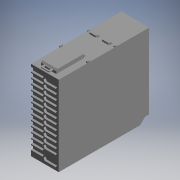
# Autodesk Inventor part: 2247681 CACN-3A-1-5
Saved by Autodesk Inventor 2017.3 (Build 213256000, 256)
## iProperties
Part Number: 2247681 CACN-3A-1-5
Material: Generic
Catalog Web Link: www.cadenas.de
Description: CACN-Power supply unit
Vendor: FESTO
Document SubType Name: Modeling
Designer: partserver
Manufacturer: FESTO
Mass: 600 g
Surface Area: 578.959 cm^2
Volume: 583.76 cm^3
Density: 1 g/cm^3
Appearance: PSOLRGB-175-175-175
Category: PARTsolutions
Company: FESTO
Title: 2247681 CACN-3A-1-5
Author: Cadenas PARTsolutions
Comments: Power supply unit
PSOL_IDENT_0: {$CADENAS_DATA\23d-libs\festo\parts\c\cacn\cacn.prj},176 {VTYP=3D},{NB=2247681 CACN-3A-1-5},{LINA=22
PSOL_IDENT_1: 47681 CACN-3A-1-5},{NN=CACN},{DATE=26.01.2021 14:46:32},{GEOMDATE=19.09.2018 12:21:51},{VERSION=},{L
PSOL_IDENT_2: INEID=50},{WBVAR=},{WBNUMERIC=}  {NB=2247681 CACN-3A-1-5},{LINA=2247681 CACN-3A-1-5},{KT=DUMMY},{TNR=
PSOL_IDENT_3: 2247681},{TYP=CACN-3A-1-5},{A=40.000},{B=130.000},{C=115.000},{VERS=1.000},{CNSMASSEXACT=0.600}
NB: 2247681 CACN-3A-1-5
NN: CACN
NT: Power supply unit
NBSYN: $TNR. $TYP.
LINA: 2247681 CACN-3A-1-5
CATALOG: Festo
TNR: 2247681
TYP: CACN-3A-1-5
A: 40
B: 130
C: 115
CNSMASSEXACT: 0.6
SUPPLIER: FESTO
ARTICLENO: 2247681 CACN-3A-1-5
BOMINFO: 2247681 CACN-3A-1-5
CREATOR: CADENAS GmbH
Autodesk Inventor part; units mm, degrees
ref_plane "YZ Plane" through (0, 0, 0) normal (1, 0, 0) x (0, 1, 0)
ref_plane "XZ Plane" through (0, 0, 0) normal (0, 1, 0) x (-1, 0, 0)
ref_plane "XY Plane" through (0, 0, 0) normal (0, 0, 1) x (1, 0, 0)
sketch "Sketch_1" plane through (0, 0, 0) normal (1, 0, 0) x (0, 1, 0)
  line L0 (52, 115) -> (-65, 115)
  line L1 (-65, 115) -> (-65, 0)
  line L2 (-65, 0) -> (-24, 0)
  line L3 (-24, 0) -> (-24, -2)
  line L4 (-24, -2) -> (-20, -2)
  line L5 (-20, -2) -> (-20, 0)
  line L6 (-20, 0) -> (15.7, 0)
  line L7 (15.7, 0) -> (15.7, -1.36)
  line L8 (15.7, -1.36) -> (18.8, -1.36)
  line L9 (18.8, -1.36) -> (18.8, 0)
  line L10 (18.8, 0) -> (65, 0)
  line L11 (65, 0) -> (65, 108)
  line L12 (65, 108) -> (59, 108)
  line L13 (59, 108) -> (52, 115)
  constraints: 28 end point
extrude "Extrusion1" add sketch "Sketch_1" along normal mid plane 40
sketch "Sketch_2" plane through (0, 0, 0) normal (1, 0, 0) x (0, 1, 0)
  line L0 (-59.6, 3) -> (-59.6, -2.3)
  line L1 (-59.6, -2.3) -> (-65.1, -2.3)
  line L2 (-65.1, -2.3) -> (-65.1, -3.3)
  line L3 (-65.1, -3.3) -> (-59.6, -3.3)
  line L4 (-59.6, -3.3) -> (-57.6, -5.3)
  line L5 (-57.6, -5.3) -> (-20.9073, -5.3)
  arc A0 (-20.9073, -5.3) -> (-20.151, -4.9542) centre (-20.9073, -4.3) ccw
  line L6 (-20.151, -4.9542) -> (-17.3487, -1.7146)
  arc A1 (-17.3487, -1.7146) -> (-17.3, -1.5838) centre (-17.5, -1.5838) ccw
  line L7 (-17.3, -1.5838) -> (-17.3, -1.4748)
  arc A2 (-17.3, -1.4748) -> (-17.473, -1.2766) centre (-17.5, -1.4748) ccw
  line L8 (-17.473, -1.2766) -> (-19.5, -1)
  line L9 (-19.5, -1) -> (-19.5, 0)
  line L10 (-19.5, 0) -> (15.7, 0)
  line L11 (15.7, 0) -> (15.7, -0.85)
  arc A3 (15.11, -1.18) -> (15.7, -0.85) centre (14.9456, -0.1936) ccw
  line L12 (15.11, -1.18) -> (12.47, -1.6455)
  line L13 (12.47, -1.6455) -> (12.8173, -3.6151)
  line L14 (12.8173, -3.6151) -> (15.42, -3.1562)
  arc A4 (15.42, -3.1562) -> (17.71, -1.36) centre (14.9459, -0.1939) ccw
  line L15 (17.71, -1.36) -> (18.8, -1.36)
  line L16 (18.8, -1.36) -> (18.8, 3)
  line L17 (18.8, 3) -> (-59.6, 3)
  constraints: 36 end point, 10 point on circle, 5 centre point
extrude "Extrusion2" add sketch "Sketch_2" along normal mid plane 27
sketch "Sketch_3" plane through (0, 0, 0) normal (0, 0, 1) x (1, 0, 0)
  line L0 (-18, 25) -> (-18, -70)
  line L1 (-18, -70) -> (19, -70)
  line L2 (19, -70) -> (19, 25)
  line L3 (19, 25) -> (-18, 25)
  line L4 (4.65, 20) -> (4.65, 11)
  line L5 (4.65, 11) -> (13.5, 11)
  line L6 (13.5, 11) -> (13.5, 20)
  line L7 (13.5, 20) -> (4.65, 20)
  line L8 (-11, -14.6) -> (-11, -59.6)
  line L9 (-11, -59.6) -> (-6.5, -59.6)
  line L10 (-6.5, -59.6) -> (-6.5, -64.1)
  line L11 (-6.5, -64.1) -> (-5.5, -65.1)
  line L12 (-5.5, -65.1) -> (5.5, -65.1)
  line L13 (5.5, -65.1) -> (6.5, -64.1)
  line L14 (6.5, -64.1) -> (6.5, -59.6)
  line L15 (6.5, -59.6) -> (11, -59.6)
  line L16 (11, -59.6) -> (11, -14.6)
  line L17 (11, -14.6) -> (-11, -14.6)
  line L18 (-13.5, 20) -> (-13.5, 11)
  line L19 (-13.5, 11) -> (-4.65, 11)
  line L20 (-4.65, 11) -> (-4.65, 20)
  line L21 (-4.65, 20) -> (-13.5, 20)
  constraints: 44 end point
extrude "Extrusion3" cut sketch "Sketch_3" against normal blind 8
sketch "Sketch_4" plane through (0, 0, 0) normal (0, 0, 1) x (1, 0, 0)
  line L0 (-4, -60.6) -> (-4, -63.1)
  line L1 (-4, -63.1) -> (4, -63.1)
  line L2 (4, -63.1) -> (4, -60.6)
  line L3 (4, -60.6) -> (-4, -60.6)
  constraints: 8 end point
extrude "Extrusion4" cut sketch "Sketch_4" against normal blind 8
sketch "Sketch_5" plane through (0, 0, 115) normal (0, 0, 1) x (1, 0, 0)
  line L0 (-13.9, 48.5) -> (-13.9, 21)
  line L1 (-13.9, 21) -> (0.4, 21)
  line L2 (0.4, 21) -> (0.4, 48.5)
  line L3 (0.4, 48.5) -> (-13.9, 48.5)
  constraints: 8 end point
extrude "Extrusion5" cut sketch "Sketch_5" against normal blind 3
sketch "Sketch_7" plane through (0, 0, 115) normal (0, 0, 1) x (1, 0, 0)
  line L0 (-13.9, -23.5) -> (-13.9, -48.5)
  line L1 (-13.9, -48.5) -> (0.4, -48.5)
  line L2 (0.4, -48.5) -> (0.4, -23.5)
  line L3 (0.4, -23.5) -> (-13.9, -23.5)
  constraints: 8 end point
sketch "Sketch7" plane through (-20, -65, 115) normal (0, 0, 1) x (1, 0, 0)
  point P0 (11.7, 77.5)
hole "Hole1" at (-8.3, 12.5, 115) direction (0, 0, -1) diameter 4 depth 3
extrude "Extrusion6" cut sketch "Sketch_7" against normal blind 3
sketch "Sketch8" plane through (-20, -65, 115) normal (0, 0, 1) x (1, 0, 0)
  point P0 (11.7, 67.5)
hole "Hole2" at (-8.3, 2.5, 115) direction (0, 0, -1) diameter 4 depth 3
sketch "Sketch_9" plane through (0, 0, 115) normal (0, 0, 1) x (1, 0, 0)
  arc A0 (-19, -63.5) -> (-18.5, -64) centre (-18.5, -63.5) ccw
  line L0 (-18.5, -64) -> (18.5, -64)
  arc A1 (18.5, -64) -> (19, -63.5) centre (18.5, -63.5) ccw
  line L1 (19, -63.5) -> (19, 50.5)
  arc A2 (19, 50.5) -> (18.5, 51) centre (18.5, 50.5) ccw
  line L2 (18.5, 51) -> (-18.5, 51)
  arc A3 (-18.5, 51) -> (-19, 50.5) centre (-18.5, 50.5) ccw
  line L3 (-19, 50.5) -> (-19, -63.5)
  circle A4 centre (-8.3, 2.5) radius 2
  circle A5 centre (-8.3, 12.5) radius 2
  line L4 (-14.4, 49) -> (-14.4, 20.5)
  line L5 (-14.4, 20.5) -> (0.65, 20.5)
  line L6 (0.65, 20.5) -> (0.65, 49)
  line L7 (0.65, 49) -> (-14.4, 49)
  line L8 (-14.4, -23) -> (-14.4, -49)
  line L9 (-14.4, -49) -> (0.65, -49)
  line L10 (0.65, -49) -> (0.65, -23)
  line L11 (0.65, -23) -> (-14.4, -23)
  constraints: 24 end point, 8 point on circle, 6 centre point
extrude "Extrusion7" add sketch "Sketch_9" along normal blind 0.2
sketch "Sketch_10" plane through (0, 0, 112) normal (0, 0, 1) x (1, 0, 0)
  circle A0 centre (-8.3, 12.5) radius 1.5
  constraints: 1 centre point
extrude "Extrusion8" add sketch "Sketch_10" along normal blind 3.5
sketch "Sketch_11" plane through (0, 21, 0) normal (0, 1, 0) x (1, 0, 0)
  arc A0 (-13.9, -114.1) -> (-12.4, -115.6) centre (-12.4, -114.1) ccw
  line L0 (-12.4, -115.6) -> (0, -115.6)
  arc A1 (0, -115.6) -> (0.4, -115.2) centre (0, -115.2) ccw
  line L1 (0.4, -115.2) -> (0.4, -112)
  line L2 (0.4, -112) -> (-13.9, -112)
  line L3 (-13.9, -112) -> (-13.9, -114.1)
  constraints: 8 end point, 4 point on circle, 2 centre point
extrude "Extrusion9" add sketch "Sketch_11" along normal blind 27.5
sketch "Sketch_12" plane through (0, 46, 0) normal (0, 1, 0) x (1, 0, 0)
  line L0 (-11, -110.5) -> (-11, -115.6)
  line L1 (-11, -115.6) -> (-4.6, -115.6)
  line L2 (-4.6, -115.6) -> (-6.85, -111.7029)
  line L3 (-6.85, -111.7029) -> (-6.85, -110.5)
  line L4 (-6.85, -110.5) -> (-11, -110.5)
  constraints: 10 end point
extrude "Extrusion10" cut sketch "Sketch_12" along normal mid plane 4
pattern_linear "Rectangular Pattern1" count 5 spacing 5 along (0, -1, 0) of "Extrusion10"
sketch "Sketch_13" plane through (0, 0, 115.6) normal (0, 0, 1) x (1, 0, 0)
  circle A0 centre (-1.9, 45.75) radius 1.8
  constraints: 1 centre point
extrude "Extrusion11" cut sketch "Sketch_13" along normal mid plane 6
pattern_linear "Rectangular Pattern2" count 5 spacing 5 along (0, -1, 0) of "Extrusion11"
sketch "Sketch_16" plane through (0, -48.5, 0) normal (0, 1, 0) x (1, 0, 0)
  arc A0 (-13.9, -114.1) -> (-12.4, -115.6) centre (-12.4, -114.1) ccw
  line L0 (-12.4, -115.6) -> (0, -115.6)
  arc A1 (0, -115.6) -> (0.4, -115.2) centre (0, -115.2) ccw
  line L1 (0.4, -115.2) -> (0.4, -112)
  line L2 (0.4, -112) -> (-13.9, -112)
  line L3 (-13.9, -112) -> (-13.9, -114.1)
  constraints: 8 end point, 4 point on circle, 2 centre point
extrude "Extrusion12" add sketch "Sketch_16" along normal blind 25
sketch "Sketch_17" plane through (0, -28.5, 0) normal (0, 1, 0) x (1, 0, 0)
  line L0 (-11, -110.5) -> (-11, -115.6)
  line L1 (-11, -115.6) -> (-4.6, -115.6)
  line L2 (-4.6, -115.6) -> (-6.85, -111.7029)
  line L3 (-6.85, -111.7029) -> (-6.85, -110.5)
  line L4 (-6.85, -110.5) -> (-11, -110.5)
  constraints: 10 end point
extrude "Extrusion13" cut sketch "Sketch_17" along normal mid plane 4
pattern_linear "Rectangular Pattern3" count 3 spacing 7.5 along (0, -1, 0) of "Extrusion13"
sketch "Sketch16" plane through (-12.4, -48.5, 115.6) normal (0, 0, 1) x (1, 0, 0)
  point P0 (10.5, 19.75)
hole "Hole3" at (-1.9, -28.75, 115.6) direction (0, 0, -1) diameter 3.6 depth 3
pattern_linear "Rectangular Pattern4" count 3 spacing 7.5 along (0, -1, 0) of "Hole3"
sketch "Sketch_21" plane through (0, 65, 0) normal (0, 1, 0) x (1, 0, 0)
  line L0 (-17.567, -10.5) -> (-15.8349, -13.5)
  line L1 (-15.8349, -13.5) -> (0.2009, -13.5)
  line L2 (0.2009, -13.5) -> (1.933, -10.5)
  line L3 (1.933, -10.5) -> (0.2009, -7.5)
  line L4 (0.2009, -7.5) -> (-15.8349, -7.5)
  line L5 (-15.8349, -7.5) -> (-17.567, -10.5)
  constraints: 12 end point
extrude "Extrusion14" cut sketch "Sketch_21" against normal blind 3
pattern_linear "Rectangular Pattern5" count 11 spacing 7.5 along (0, 0, 1) of "Extrusion14"
sketch "Sketch_25" plane through (0, 65, 0) normal (0, 1, 0) x (1, 0, 0)
  line L0 (-17.567, -100.5) -> (-15.8349, -103.5)
  line L1 (-15.8349, -103.5) -> (0.2009, -103.5)
  line L2 (0.2009, -103.5) -> (1.933, -100.5)
  line L3 (1.933, -100.5) -> (0.2009, -97.5)
  line L4 (0.2009, -97.5) -> (-15.8349, -97.5)
  line L5 (-15.8349, -97.5) -> (-17.567, -100.5)
  constraints: 12 end point
extrude "Extrusion15" cut sketch "Sketch_25" against normal blind 3
sketch "Sketch_26" plane through (0, 65, 0) normal (0, 1, 0) x (1, 0, 0)
  line L0 (1.4, -6.75) -> (3.1321, -9.75)
  line L1 (3.1321, -9.75) -> (20, -9.75)
  line L2 (20, -9.75) -> (20, -3.75)
  line L3 (20, -3.75) -> (3.1321, -3.75)
  line L4 (3.1321, -3.75) -> (1.4, -6.75)
  constraints: 10 end point
extrude "Extrusion16" cut sketch "Sketch_26" against normal blind 3
pattern_linear "Rectangular Pattern6" count 13 spacing 7.5 along (0, 0, 1) of "Extrusion16"
sketch "Sketch_22" plane through (0, -62, 0) normal (0, 1, 0) x (1, 0, 0)
  line L0 (-17.567, -10.5) -> (-15.8349, -13.5)
  line L1 (-15.8349, -13.5) -> (0.2009, -13.5)
  line L2 (0.2009, -13.5) -> (1.933, -10.5)
  line L3 (1.933, -10.5) -> (0.2009, -7.5)
  line L4 (0.2009, -7.5) -> (-15.8349, -7.5)
  line L5 (-15.8349, -7.5) -> (-17.567, -10.5)
  constraints: 12 end point
extrude "Extrusion17" cut sketch "Sketch_22" against normal blind 3
pattern_linear "Rectangular Pattern7" count 12 spacing 7.5 along (0, 0, 1) of "Extrusion17"
sketch "Sketch_28" plane through (0, -62, 0) normal (0, 1, 0) x (1, 0, 0)
  line L0 (-17.567, -108) -> (-15.8349, -111)
  line L1 (-15.8349, -111) -> (0.2009, -111)
  line L2 (0.2009, -111) -> (1.933, -108)
  line L3 (1.933, -108) -> (0.2009, -105)
  line L4 (0.2009, -105) -> (-15.8349, -105)
  line L5 (-15.8349, -105) -> (-17.567, -108)
  constraints: 12 end point
extrude "Extrusion18" cut sketch "Sketch_28" against normal blind 3
sketch "Sketch_29" plane through (0, -62, 0) normal (0, 1, 0) x (1, 0, 0)
  line L0 (1.4, -6.75) -> (3.1321, -9.75)
  line L1 (3.1321, -9.75) -> (20, -9.75)
  line L2 (20, -9.75) -> (20, -3.75)
  line L3 (20, -3.75) -> (3.1321, -3.75)
  line L4 (3.1321, -3.75) -> (1.4, -6.75)
  constraints: 10 end point
extrude "Extrusion19" cut sketch "Sketch_29" against normal blind 3
pattern_linear "Rectangular Pattern8" count 14 spacing 7.5 along (0, 0, 1) of "Extrusion19"
ref_plane "LINKS_XY" through (-20, 0, 0) normal (1, 0, 0) x (0, 1, 0)
ref_plane "LINKS_YZ" through (-20, 0, 0) normal (0, 1, 0) x (0, 0, 1)
ref_plane "LINKS_ZX" through (-20, 0, 0) normal (0, 0, 1) x (1, 0, 0)
ref_plane "RECHTS_XY" through (20, 0, 0) normal (-1, 0, 0) x (0, 1, 0)
ref_plane "RECHTS_YZ" through (20, 0, 0) normal (0, 1, 0) x (0, 0, -1)
ref_plane "RECHTS_ZX" through (20, 0, 0) normal (0, 0, -1) x (-1, 0, 0)
body "Solid1"
